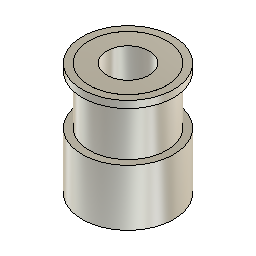
Pulley, 16 tooths, drill hole 6mm (Autodesk Fusion 360 design; units mm, degrees)
Autodesk Fusion 360 part; units mm, degrees
sketch "Skizze1" plane through (0, 0, 0) normal (0, 0, 1) x (1, 0, 0)
  circle A0 centre (0, 0) radius 6.5
  circle A1 centre (0, 0) radius 3
  dimension "d1" = 13
  dimension "d2" = 6
  constraint coincident A0.centre A1.centre
  measures "d1" diameter of A0
  measures "d2" diameter of A1
extrude "Extrusion1" add sketch "Skizze1" along normal blind 8 makes body 1
sketch "Skizze2" plane through (0, 0, 8) normal (0, 0, 1) x (-1, 0, 0)
  circle A0 centre (0, 0) radius 3
  circle A1 centre (0, 0) radius 6.5
  circle A2 centre (0, 0) radius 5.5
  dimension "d5" = 11
  constraint concentric A0 A2
  measures "d5" diameter of A2
extrude "Extrusion2" add sketch "Skizze2" along normal blind 7 contours A2 bodies 1
sketch "Skizze3" plane through (0, 0, 15) normal (0, 0, 1) x (-1, 0, 0)
  circle A0 centre (0, 0) radius 3
  circle A1 centre (0, 0) radius 5.5
  circle A2 centre (0, 0) radius 6.5
  dimension "d8" = 13
  constraint concentric A0 A2
  measures "d8" diameter of A2
extrude "Extrusion4" add sketch "Skizze3" along normal blind 1 separate body contours A2 makes body 2
extrude "Extrusion3" add sketch "Skizze3" along normal blind 1 contours A1 bodies 1
